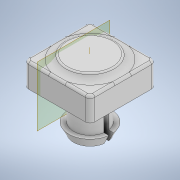
# Autodesk Inventor part: Small_Button
Saved by Autodesk Inventor 2021 (Build 250183000, 183)
## iProperties
Created: 2020-05-31
Part Number: Small_Button
Material: Generic
Document SubType Name: Modeling
Designer: ameli
Density: 1 g/cm^3
Appearance: Default
Author: ameli
Autodesk Inventor part; units mm, degrees
ref_plane "YZ Plane" through (0, 0, 0) normal (1, 0, 0) x (0, 1, 0)
ref_plane "XZ Plane" through (0, 0, 0) normal (0, 1, 0) x (-1, 0, 0)
ref_plane "XY Plane" through (0, 0, 0) normal (0, 0, 1) x (1, 0, 0)
sketch "Sketch5" plane through (0, 0, 0) normal (0, 1, 0) x (-1, 0, 0)
  line L0 (0, 0) -> (14, 0)
  line L1 (14, 0) -> (14, -14)
  line L2 (14, -14) -> (0, -14)
  line L3 (0, -14) -> (0, 0)
  dimension "d3" = 14
  dimension "d4" = 14
  constraints: 8 end point, 2 parallel, 1 horizontal, 1 perpendicular
  measures "d3" distance of L1.end L2.end
  measures "d4" distance of L0.end L1.end
extrude "Extrusion1" add sketch "Sketch5" along normal blind 5
sketch "Sketch6" plane through (0, 5, 0) normal (0, 1, 0) x (1, 0, 0)
  circle A0 centre (-7, 7) radius 5
  line L0 (0, 0) -> (0, 14) projected
  line L1 (0, 14) -> (-14, 14) projected
  dimension "d7" = 10
  dimension "d8" = 7
  dimension "d9" = 7
  constraints: 1 centre point
  measures "d7" diameter of A0
  measures "d8" distance from line of L0 A0.centre
  measures "d9" distance from line of L1 A0.centre
extrude "Extrusion2" add sketch "Sketch6" along normal blind 1
fillet "Fillet1" radius 2 1 edges at (-12, 5, -7)
fillet "Fillet2" radius 1 4 edges at (-14, 2.5, 0) (0, 2.5, 0) (-14, 2.5, -14) (0, 2.5, -14)
fillet "Fillet3" radius 0.5 9 edges at (-12, 6, -7) (-0.2929, 5, -13.7071) (-7, 5, -14) (-13.7071, 5, -13.7071) (-14, 5, -7) (-13.7071, 5, -0.2929) (-7, 5, 0) (-0.2929, 5, -0.2929) (0, 5, -7)
shell "Shell1" thickness 1.5 removed faces 1 at (-9, 0, -9.3333)
sketch "Sketch8" plane through (-7, 4.5, -7) normal (0, -1, 0) x (1, 0, 0)
  circle A0 centre (0, 0) radius 3.5
  circle A1 centre (0, 0) radius 4.2826 projected
  point P0 (7, 7)
  dimension "d16" = 7
  constraints: 1 centre point, 1 concentric
  measures "d16" diameter of A0
extrude "Extrusion3" add sketch "Sketch8" along normal blind 13 contours A0
fillet "Fillet4" radius 2 1 edges at (-10.5, 4.5, -7)
ref_plane "Work Plane2" through (-7, 0, -1) normal (1, 0, 0) x (0, 0, -1)
sketch "Sketch11" plane through (-7, 0, -1) normal (1, 0, 0) x (0, 0, -1)
  line L0 (2.5, -8.5) -> (9.5, -8.5) projected
  line L1 (9.5, -8.5) -> (10.5, -6.5)
  line L2 (9.5, -8.5) -> (11.7361, -8.5) construction
  line L3 (10.5, -6.5) -> (9.5, -6.5)
  line L4 (9.5, 2.9132) -> (9.5, -8.5) projected
  line L5 (9.5, -6.5) -> (9.5, -8.5)
  line L6 (6, 8.9) -> (6, -11.4) projected
  point P0 (-1, 0)
  dimension "d23" = 1
  dimension "d40" = 2
  constraints: 8 end point, 2 horizontal, 1 collinear, 1 equal length, 1 point on line
  measures "d23" distance of L1.end L3.end
  measures "d40" distance between parallel lines of L0 L3
revolve "Revolution1" add sketch "Sketch11" angle 360 about axis through (-7, 4.5, -7) along (0, -1, 0)
ref_plane "Work Plane3" through (-10.5, 4.5, -7) normal (-1, 0, 0) x (0, -1, 0)
sketch "Sketch17" plane through (-10.5, 4.5, -7) normal (-1, 0, 0) x (0, -1, 0)
  line L0 (13, -3.5) -> (13, 3.5) projected
  line L1 (13, 0) -> (13, 0.5)
  line L2 (13, 0.5) -> (5, 0.5)
  line L3 (5, 0.5) -> (5, -0.5)
  line L4 (5, -0.5) -> (13, -0.5)
  line L5 (13, -0.5) -> (13, 0)
  arc A0 (5, 0.5) -> (5, -0.5) centre (5, 0) ccw
  point P0 (4.5, 7)
  point P1 (13, -0.5)
  dimension "d32" = 0.5
  dimension "d33" = 8
  dimension "d34" = 1
  dimension "d35" = 8
  constraints: 10 end point, 2 midpoint, 2 perpendicular, 2 point on circle, 2 point on line, 1 centre point
  measures "d32" distance of L1.start L1.end
  measures "d33" distance of L1.end L2.end
  measures "d34" distance of L2.end L3.end
  measures "d35" distance of L3.end L4.end
extrude "Extrusion4" cut sketch "Sketch17" along normal blind 1 and the other way blind 9
body "Solid1"
